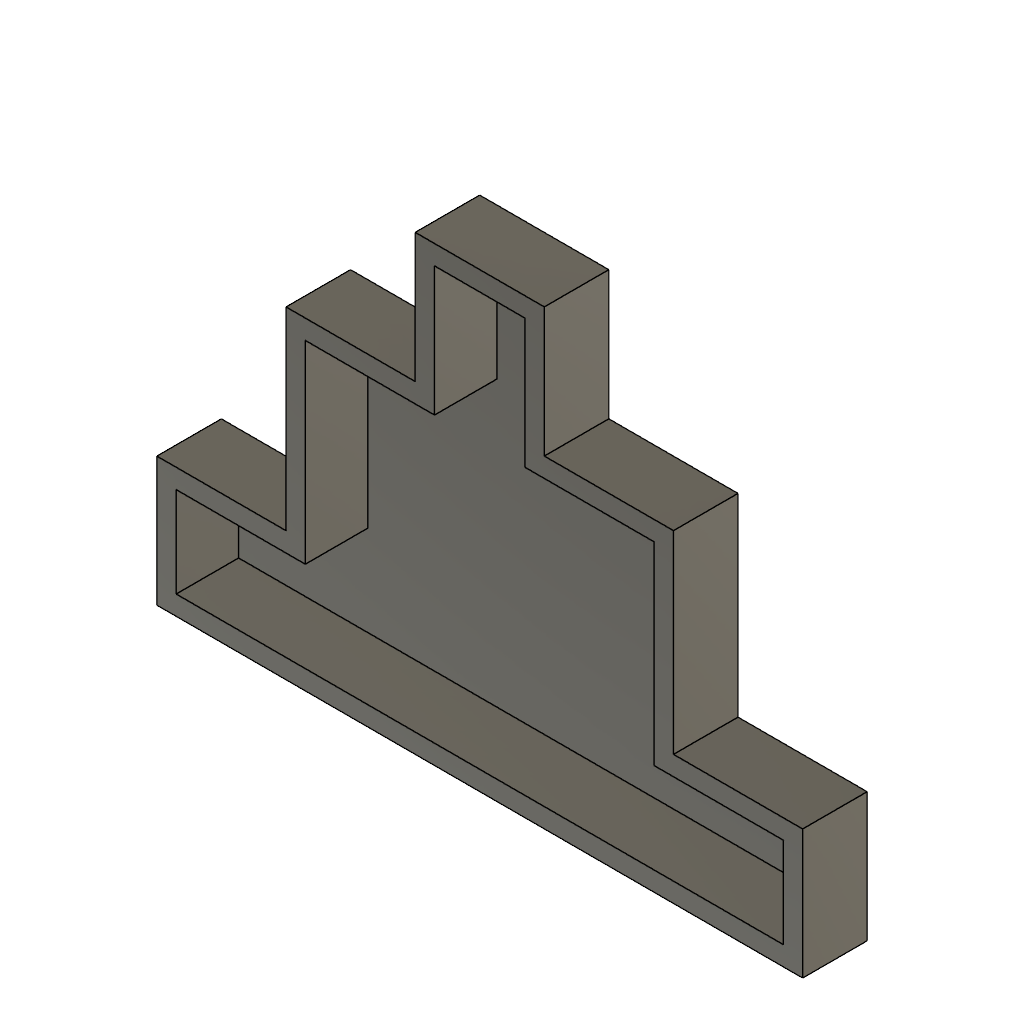
exercise 14 (Autodesk Fusion 360 design; units mm, degrees)
part number: 2026-10-07-17-33-41-261
Autodesk Fusion 360 part; units mm, degrees
sketch "Sketch1" plane through (0, 0, 0) normal (0, 1, 0) x (1, 0, 0)
  line L0 (-55.6722, 27.0003) -> (-55.6722, -2.9997)
  line L1 (-55.6722, -2.9997) -> (-25.6722, -2.9997)
  line L2 (-25.6722, -2.9997) -> (-25.6722, -47.9997)
  line L3 (-25.6722, -47.9997) -> (4.3278, -47.9997)
  line L4 (4.3278, -47.9997) -> (4.3278, -77.9997)
  line L5 (4.3278, -77.9997) -> (34.3278, -77.9997)
  line L6 (34.3278, -77.9997) -> (34.3278, -47.9997)
  line L7 (34.3278, -47.9997) -> (64.3278, -47.9997)
  line L8 (64.3278, -47.9997) -> (64.3278, -2.9997)
  line L9 (64.3278, -2.9997) -> (94.3278, -2.9997)
  line L10 (94.3278, -2.9997) -> (94.3278, 27.0003)
  line L11 (-55.6722, 27.0003) -> (94.3278, 27.0003)
  dimension "d1" = 150
  dimension "d2" = 30
  dimension "d3" = 30
  dimension "d4" = 30
  dimension "d5" = 30
  dimension "d6" = 30
  dimension "d7" = 45
  dimension "d8" = 30
  dimension "d9" = 30
  dimension "d10" = 45
  constraint vertical L0
  constraint perpendicular L0 L1
  constraint perpendicular L1 L2
  constraint perpendicular L2 L3
  constraint perpendicular L3 L4
  constraint perpendicular L4 L5
  constraint perpendicular L5 L6
  constraint perpendicular L6 L7
  constraint perpendicular L7 L8
  constraint perpendicular L8 L9
  constraint perpendicular L7 L10
  constraint perpendicular L10 L11
  measures "d1" distance of L0.start L10.end
  measures "d2" distance of L4.end L5.end
  measures "d3" horizontal distance of L2.end L4.end
  measures "d4" horizontal distance of L0.end L2.end
  measures "d5" distance of L6.end L7.end
  measures "d6" distance of L0.start L0.end
  measures "d7" vertical distance of L0.end L2.end
  measures "d8" vertical distance of L2.end L4.end
  measures "d9" distance of L5.end L6.end
  measures "d10" vertical distance of L7.end L9.end
extrude "Extrude1" add sketch "Sketch1" along normal blind 15 makes body 1
move_face "OffsetFaces1" offset -4.5 12 faces at (34.3278, 10, 67.9997) (64.3278, 10, 32.9997) (44.3278, 5, 47.9997) (74.3278, 10, 2.9997) (94.3278, 10, -7.0003) (-45.6722, 10, 2.9997) (-15.6722, 10, 47.9997) (14.3278, 10, 77.9997) (4.3278, 10, 57.9997) (-25.6722, 10, 17.9997) (-55.6722, 10, -17.0003) (-5.6722, 5, -27.0003) on bodies 1
extrude "Extrude2" add sketch "Sketch1" along normal blind 15 separate body makes body 2
extrude "Extrude3" cut 1 faces at (22.8278, 0, 13.4997) along direction (0, 1, 0) blind 14.5 on bodies 1 bodies 1 2
